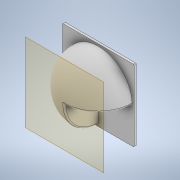
# Autodesk Inventor part: hemisephere
Saved by Autodesk Inventor 2022.3 (Build 263350000, 350)
## iProperties
Created: 2022-06-10
Part Number: hemisephere
Material: Generic
Document SubType Name: Modeling
Designer: swang
Density: 1 g/cm^3
Appearance: Default
Author: swang
Autodesk Inventor part; units mm, degrees
ref_plane "YZ Plane" through (0, 0, 0) normal (1, 0, 0) x (0, 1, 0)
ref_plane "XZ Plane" through (0, 0, 0) normal (0, 1, 0) x (-1, 0, 0)
ref_plane "XY Plane" through (0, 0, 0) normal (0, 0, 1) x (1, 0, 0)
sketch "Sketch1" plane through (0, 0, 0) normal (0, 0, 1) x (1, 0, 0)
  line L0 (-47.5, -47.5) -> (47.5, -47.5)
  line L1 (47.5, -47.5) -> (47.5, 47.5)
  line L2 (47.5, 47.5) -> (-47.5, 47.5)
  line L3 (-47.5, 47.5) -> (-47.5, -47.5)
  line L4 (-47.5, -47.5) -> (47.5, 47.5) construction
  line L5 (47.5, -47.5) -> (-47.5, 47.5) construction
  point P0 (0, 0)
  dimension "d0" = 95
  dimension "d1" = 95
  constraints: 12 end point, 2 midpoint, 2 parallel, 1 horizontal, 1 perpendicular
  measures "d0" distance of L1.end L2.end
  measures "d1" distance of L2.end L0.start
extrude "Extrusion1" add sketch "Sketch1" along normal blind 3
sketch "Sketch2" plane through (0, 0, 0) normal (0, 1, 0) x (-1, 0, 0)
  line L0 (-47.5, 3) -> (47.5, 3) projected
  line L1 (0, 48) -> (0, 3)
  line L2 (-47.5, 0) -> (47.5, 0) projected
  arc A0 (0, 48) -> (-44.8999, 0) centre (0, 3) ccw
  arc A1 (44.8999, 0) -> (45, 3) centre (0, 3) ccw
  line L3 (0, -11.5492) -> (0, 69.2892) projected
  point P0 (0, 0)
  point P1 (-45, 3)
  constraints: 4 point on circle, 3 point on line, 2 centre point, 2 end point, 1 midpoint, 1 perpendicular
revolve "Revolution1" add sketch "Sketch2" angle 360 about axis through (0, 0, -10) along (0, 0, 1) contours L0 A0 L1
fillet "Fillet1" radius 1 4 edges at (47.5, -47.5, 1.5) (47.5, 47.5, 1.5) (-47.5, -47.5, 1.5) (-47.5, 47.5, 1.5)
ref_plane "Work Plane1" through (0, 0, 48) normal (0, 0, 1) x (1, 0, 0)
sketch "Sketch3" plane through (0, 0, 48) normal (0, 0, 1) x (1, 0, 0)
  line L0 (0, 0) -> (47.5, 0)
  line L1 (47.5, 0) -> (47.5, -47.6383)
  line L2 (47.5, -47.6383) -> (0, -47.6383)
  line L3 (0, -47.6383) -> (0, 0)
  constraints: 8 end point, 2 parallel, 1 horizontal, 1 perpendicular
extrude "Extrusion2" cut sketch "Sketch3" against normal up to surface (45 mm away)
fillet "Fillet2" radius 2 2 edges at (0, -31.8198, 34.8198) (31.8198, 0, 34.8198)
sketch "Sketch5" plane through (0, 0, 0) normal (0, 0, -1) x (-1, 0, 0)
  line L0 (0, 0) -> (-42.9535, 0) projected
  circle A0 centre (0, 0) radius 15
  dimension "d11" = 30
  constraints: 1 centre point, 1 coincident
  measures "d11" diameter of A0
extrude "Extrusion3" add sketch "Sketch5" along normal blind 20
shell "Shell2" thickness 3 removed faces 1 at (4.8547, 1.1966, -20)
body "Solid1"
